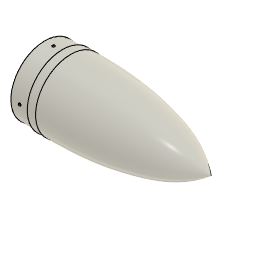
Haack Cone v2 v5 (Autodesk Fusion 360 design; units mm, degrees)
Autodesk Fusion 360 part; units mm, degrees
note: some values were not read from the file. Set by a fixed rule: which sketch regions a step uses.
sketch "Sketch7" plane through (0, 0, 0) normal (0, 0, 1) x (1, 0, 0)
  spline S0 degree 5 poles (152.4, 0) (151.2937, 0.9222) (149.0727, 2.7286) (145.7158, 5.3236) (141.1893, 8.5541) (135.4464, 12.2085) (129.6198, 15.4814) (123.7124, 18.3823) (117.7301, 20.9309) (111.683, 23.1627) (105.5843, 25.1244) (99.4482, 26.8665) (93.2881, 28.4361) (87.1148, 29.8711) (80.9343, 31.1911) (74.7482, 32.4005) (68.5558, 33.4944) (62.3548, 34.464) (56.1435, 35.3022) (49.9217, 36.0094) (43.6907, 36.5932) (37.4529, 37.0648) (31.2109, 37.437) (24.9673, 37.7217) (18.7236, 37.9276) (12.4808, 38.0603) (7.4877, 38.1105) (3.7436, 38.1172) (1.2478, 38.108) (0, 38.1) knots 0 0 0 0 0 0 0.04 0.08 0.12 0.16 0.2 0.24 0.28 0.32 0.36 0.4 0.44 0.48 0.52 0.56 0.6 0.64 0.68 0.72 0.76 0.8 0.84 0.88 0.92 0.96 1 1 1 1 1 1
  line L0 (152.4, 0) -> (-50.8, 0)
  line L1 (143.7999, 0.3384) -> (145.9125, -1.2855)
  line L2 (-8.9994, 38.1) -> (0, 38.1)
  line L3 (-2.9994, 38.1) -> (3.0006, 38.1)
  spline S1 degree 3 poles (151.7597, -0.7681) (143.553, 6.0732) (135.0733, 11.6208) (126.327, 15.9341) (116.3141, 20.872) (105.9326, 24.1777) (95.4388, 26.8364) (87.0315, 28.9664) (78.5762, 30.7296) (70.1161, 32.1847) (59.9964, 33.9253) (49.841, 35.1306) (39.6462, 35.8822) (27.2551, 36.7958) (14.8313, 37.1373) (2.4257, 37.1104) (1.6192, 37.1087) (0.8128, 37.1052) (0.0064, 37.1) knots 0 0 0 0 0.179235 0.179235 0.179235 0.384426 0.384426 0.384426 0.548818 0.548818 0.548818 0.74546 0.74546 0.74546 0.984463 0.984463 0.984463 1 1 1 1
  line L4 (-8.9994, 38.1) -> (-14.9994, 38.1) construction
  line L5 (-8.9994, 38.1) -> (-8.9994, 36.83)
  line L6 (-8.9994, 36.83) -> (-28.0494, 36.83)
  line L7 (-28.0494, 36.83) -> (-28.0494, 35.83)
  line L8 (-28.0494, 35.83) -> (-8.9994, 35.83)
  line L9 (-8.9994, 35.83) -> (0.0064, 37.1)
  point P0 (121.92, 19.0912)
  point P1 (91.44, 28.8463)
  point P2 (60.96, 34.6306)
  point P3 (30.48, 37.453)
  dimension "d16" = -1
  dimension "d31" = 1.27
  dimension "d32" = 19.05
  dimension "d39" = 1
  constraint coincident L2 L3.start
  constraint perpendicular L5 L6
  constraint vertical L7
  constraint perpendicular L7 L8
  measures "d31" distance of L2.start L5.end
  measures "d32" distance of L5.end L6.end
  measures "d39" distance of L6.end L7.end
revolve "Revolve4" add sketch "Sketch7" angle 360 about axis through (1.75, 0, 0) along (1, 0, 0)
ref_plane "WorkPlane5" through (-19.133, 36.83, 0) normal (0, 1, 0) x (0, 0, -1)
sketch "Sketch12" plane through (0, 36.83, 0) normal (0, 1, 0) x (1, 0, 0)
  line L0 (-8.9994, 0) -> (-18.5244, 0) construction
  circle A0 centre (-18.5244, 0) radius 1.5
  point P0 (-8.9994, 0)
  dimension "d41" = 9.525
  dimension "d42" = 3
  constraint coincident P0 L0.start
  constraint horizontal L0
  constraint coincident L0.end A0.centre
  measures "d41" distance of P0 L0.end
  measures "d42" diameter of A0
ref_plane "WorkPlane6" through (-19.0893, 0, 36.83) normal (0, 0, 1) x (0, 1, 0)
sketch "Sketch13" plane through (0, 0, 36.83) normal (0, 0, 1) x (1, 0, 0)
  line L0 (-8.9994, -36.83) -> (-8.9994, 36.83)
  line L1 (-28.0494, -36.83) -> (-28.0494, 36.83)
  line L2 (-8.9994, 0) -> (-18.5244, 0) construction
  circle A0 centre (-18.5244, 0) radius 1.5
  dimension "d44" = 9.525
  dimension "d45" = 3
  constraint midpoint L0 L2.start
  constraint perpendicular L1 L2
  constraint coincident L2.end A0.centre
  measures "d44" distance of L2.start L2.end
  measures "d45" diameter of A0
extrude "Extrude6" cut sketch "Sketch13" against normal blind 96.52
extrude "Extrude7" cut sketch "Sketch12" against normal blind 91.44
